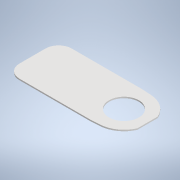
# Autodesk Inventor part: Laser-Pivot-Ringpull
Saved by Autodesk Inventor 2021 (Build 250183000, 183)
## iProperties
Created: 2020-07-21
Part Number: Laser-Pivot-Ringpull
Material: Generic
Document SubType Name: Modeling
Designer: lucas
Density: 1 g/cm^3
Appearance: Default
Project: 4Wire-Laser
Author: lucas
Revision Number: RLS_001
Autodesk Inventor part; units mm, degrees
ref_plane "YZ Plane" through (0, 0, 0) normal (1, 0, 0) x (0, 1, 0)
ref_plane "XZ Plane" through (0, 0, 0) normal (0, 1, 0) x (-1, 0, 0)
ref_plane "XY Plane" through (0, 0, 0) normal (0, 0, 1) x (1, 0, 0)
sketch "Sketch1" plane through (0, 0, 0) normal (0, 1, 0) x (-1, 0, 0)
  circle A0 centre (0, 0) radius 5.7
  arc A1 (0, 9) -> (0, -9) centre (0, 0) ccw construction
  line L0 (0, 9) -> (12.65, 9) construction
  line L1 (12.65, 9) -> (12.65, -9) construction
  line L2 (0, 0) -> (0, -9) construction
  line L3 (3.0786, -10) -> (30, -10)
  line L4 (35, -5) -> (35, 5)
  line L5 (30, 10) -> (3.0786, 10)
  arc A2 (35, 5) -> (30, 10) centre (30, 5) ccw
  arc A3 (30, -10) -> (35, -5) centre (30, -5) ccw
  line L6 (2.8334, -9.9925) -> (-0.6007, -9.7816)
  line L7 (2.8334, 9.9925) -> (-0.6007, 9.7816)
  arc A4 (2.8334, -9.9925) -> (3.0786, -10) centre (3.0786, -6) ccw
  arc A5 (3.0786, 10) -> (2.8334, 9.9925) centre (3.0786, 6) ccw
  line L8 (0, 0) -> (36.2824, 0)
  line L9 (-9, 3.8781) -> (-9, -3.8781)
  arc A6 (-0.6007, 9.7816) -> (-9, 3.8781) centre (0, 0) ccw
  arc A7 (-9, -3.8781) -> (-0.6007, -9.7816) centre (0, 0) ccw
  point P0 (35, -10)
  point P1 (35, 10)
  point P2 (2, -10)
  point P3 (2.9559, 10)
  dimension "d0" = 11.4
  dimension "d1" = 9
  dimension "d2" = 12.65
  dimension "d6" = 5
  dimension "d10" = 20
  dimension "d12" = 4
  dimension "d13" = 20
  dimension "d14" = 20
  constraints: 20 end point, 14 point on circle, 10 tangent, 8 centre point, 7 point on line, 3 coincident, 3 horizontal, 3 perpendicular, 3 vertical, 2 equal radius
  measures "d0" diameter of A0
  measures "d1" radius of A1
  measures "d2" distance of L0.start L0.end
  measures "d6" radius of A2
  measures "d10" distance between parallel lines of L5 L3
  measures "d12" radius of A4
  measures "d13" diameter of L5 L8
  measures "d14" diameter of L3 L8
extrude "Extrusion1" add sketch "Sketch1" along normal blind 0.5
body "Solid1"
